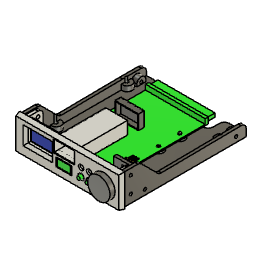
Gotek Case v24 (Autodesk Fusion 360 design; units mm, degrees)
Autodesk Fusion 360 part; units mm, degrees
(part 1 of 2)
sketch "Sketch1" plane through (0, 0, 0) normal (0, 0, 1) x (1, 0, 0)
  line L0 (-75, 0) -> (-75, 112)
  line L1 (-75, 112) -> (-134, 112)
  line L2 (-134, 112) -> (-134, 47.5)
  line L3 (-75, 0) -> (-114, 0)
  line L4 (-114, 0) -> (-114, 47.5)
  line L5 (-134, 47.5) -> (-114, 47.5)
  circle A0 centre (-79.5, 88.5) radius 1.5
  circle A1 centre (-129.5, 88.5) radius 1.5
  circle A2 centre (-79.5, 67.5) radius 1.5
  circle A3 centre (-129.5, 67.5) radius 1.5
  circle A4 centre (-79.5, 17.5) radius 1.5
  dimension "d1" = 112
  dimension "d2" = 59
  dimension "d3" = 64.5
  dimension "d4" = 39
  dimension "d11" = 3
  dimension "d12" = 3
  dimension "d13" = 3
  dimension "d14" = 3
  dimension "d15" = 3
  constraint vertical L0
  constraint perpendicular L0 L1
  constraint perpendicular L1 L2
  constraint perpendicular L0 L3
  constraint perpendicular L3 L4
  constraint perpendicular L4 L5
  measures "d1" distance of L0.start L0.end
  measures "d2" distance of L0.end L1.end
  measures "d3" distance of L1.end L2.end
  measures "d4" distance of L0.start L3.end
  measures "d11" diameter of A0
  measures "d12" diameter of A1
  measures "d13" diameter of A2
  measures "d14" diameter of A3
  measures "d15" diameter of A4
extrude "Extrude1" add sketch "Sketch1" along normal blind 1.1 makes body 1
box "BoxPrimitive1" add length 6 width 15 height 7 placed x (0, 1, 0) y (-1, 0, 0) z (0, 0, 1) at (-76, 2, 1.1) bodies 1
sketch "Sketch3" plane through (0, 2, 0) normal (0, -1, 0) x (1, 0, 0)
  line L0 (-91, 8.1) -> (-91, 1.1)
  line L1 (-91, 1.1) -> (-76, 1.1)
  line L2 (-76, 1.1) -> (-76, 8.1)
  line L3 (-76, 8.1) -> (-91, 8.1)
  circle A0 centre (-87.5, 5.1) radius 1.75
  circle A1 centre (-79.5, 5.1) radius 1.75
  dimension "d25" = 3.5
  dimension "d26" = 3.5
  measures "d25" diameter of A0
  measures "d26" diameter of A1
extrude "Extrude2" add sketch "Sketch3" along normal blind 5.5 contours A0 | A1 bodies 1
sketch "Sketch4" plane through (0, 0, 1.1) normal (0, 0, 1) x (-1, 0, 0)
  line L0 (76, -8) -> (76, -2)
  line L1 (76, -2) -> (91, -2)
  line L2 (91, -2) -> (91, -8)
  line L3 (91, -8) -> (76, -8)
  circle A0 centre (79.5, -88.5) radius 1.5
  circle A1 centre (129.5, -67.5) radius 1.5
  circle A2 centre (79.5, -67.5) radius 1.5
  circle A3 centre (129.5, -88.5) radius 1.5
  circle A4 centre (79.5, -17.5) radius 1.5
  line L4 (75, 0) -> (75, -112)
  line L5 (75, -112) -> (134, -112)
  line L6 (134, -112) -> (134, -47.5)
  line L7 (134, -47.5) -> (114, -47.5)
  line L8 (114, -47.5) -> (114, 0)
  line L9 (114, 0) -> (75, 0)
  line L10 (97.5, 1) -> (111.5, 1)
  line L11 (111.5, 1) -> (111.5, -13)
  line L12 (111.5, -13) -> (97.5, -13)
  line L13 (97.5, -13) -> (97.5, 1)
  dimension "d31" = 14
  dimension "d32" = 14
  constraint horizontal L10
  constraint vertical L11
  constraint horizontal L12
  constraint vertical L13
  measures "d31" distance of L10.start L10.end
  measures "d32" distance of L10.start L12.end
extrude "Extrude3" add sketch "Sketch4" along normal blind 8 contours L9 L10 L11 L13 | L9 L11 L12 L13 bodies 1
box "BoxPrimitive2" add length 3 width 59 height 5 placed x (0, -1, 0) y (1, 0, 0) z (0, 0, 1) at (-134, 112, 1.1) bodies 1
sketch "Sketch6" plane through (0, 112, 0) normal (0, 1, 0) x (-1, 0, 0)
  line L0 (75, 0) -> (134, 0)
  line L1 (134, 0) -> (134, 6.1)
  line L2 (134, 6.1) -> (75, 6.1)
  line L3 (75, 6.1) -> (75, 0)
  line L4 (76.25, 1.25) -> (132.75, 1.25)
  line L5 (132.75, 1.25) -> (132.75, 4.85)
  line L6 (132.75, 4.85) -> (76.25, 4.85)
  line L7 (76.25, 4.85) -> (76.25, 1.25)
  dimension "d40" = -1.25
extrude "Extrude4" add sketch "Sketch6" along normal blind 8 contours L4 L5 L6 L7 bodies 1
sketch "Sketch10" plane through (0, 0, 0) normal (0, 1, 0) x (1, 0, 0)
  line L0 (-200, -10) -> (-212, -10)
  line L1 (-212, -10) -> (-212, -24)
  line L2 (-212, -24) -> (-200, -24)
  line L3 (-200, -24) -> (-200, -10)
  dimension "d65" = 12
  dimension "d66" = 14
  constraint horizontal L0
  constraint vertical L1
  constraint horizontal L2
  constraint vertical L3
  measures "d65" distance of L0.start L0.end
  measures "d66" distance of L0.start L2.end
extrude "Extrude8" add sketch "Sketch10" along normal blind 6 separate body makes body 2
cylinder "CylinderPrimitive1" add diameter 7 height 7.5 placed x (1, 0, 0) y (0, 0, 1) z (0, -1, 0) at (-206, 0, 17) bodies 2
cylinder "CylinderPrimitive2" add diameter 4 height 1 placed x (1, 0, 0) y (0, 0, 1) z (0, -1, 0) at (-206, -7.5, 17) bodies 2
cylinder "CylinderPrimitive3" add diameter 6 height 12.5 placed x (1, 0, 0) y (0, 0, 1) z (0, -1, 0) at (-206, -8.5, 17) bodies 2
sketch "Sketch14" plane through (0, -21, 0) normal (0, -1, 0) x (1, 0, 0)
  circle A0 centre (-206, 17) radius 3
  line L0 (-209.5054, 18.5) -> (-202.5, 18.5)
  line L1 (-202.5, 18.5) -> (-202.5, 20.3)
  line L2 (-202.5, 20.3) -> (-209.5054, 20.3)
  line L3 (-209.5054, 20.3) -> (-209.5054, 18.5)
  constraint horizontal L0
  constraint vertical L1
  constraint horizontal L2
  constraint vertical L3
extrude "Extrude9" cut sketch "Sketch14" against normal blind 12 contours A0 L0 | A0 L0 L1 L2 L3 picked at (-205.8141, 19.2331) bodies 2
sketch "Sketch15" plane through (0, 0, 24) normal (0, 0, 1) x (-1, 0, 0)
  line L0 (212, 0) -> (200, 0)
  line L1 (200, 0) -> (200, -6)
  line L2 (200, -6) -> (212, -6)
  line L3 (212, -6) -> (212, 0)
  line L4 (209.29, -6) -> (207.79, -6)
  line L5 (207.79, -6) -> (207.79, -3)
  line L6 (207.79, -3) -> (209.29, -3)
  line L7 (209.29, -3) -> (209.29, -6)
  line L8 (209.29, -6) -> (207.79, -3) construction
  line L9 (207.79, -6) -> (209.29, -3) construction
  line L10 (202.71, -6) -> (204.21, -6)
  line L11 (204.21, -6) -> (204.21, -3)
  line L12 (204.21, -3) -> (202.71, -3)
  line L13 (202.71, -3) -> (202.71, -6)
  line L14 (202.71, -6) -> (204.21, -3) construction
  line L15 (204.21, -6) -> (202.71, -3) construction
  line L16 (206.75, -6) -> (205.25, -6)
  line L17 (205.25, -6) -> (205.25, -3)
  line L18 (205.25, -3) -> (206.75, -3)
  line L19 (206.75, -3) -> (206.75, -6)
  line L20 (206.75, -6) -> (205.25, -3) construction
  line L21 (205.25, -6) -> (206.75, -3) construction
  point P0 (208.54, -4.5)
  point P1 (203.46, -4.5)
  point P2 (206, -4.5)
  dimension "d82" = 1.5
  dimension "d83" = 1.5
  dimension "d84" = 1.5
  constraint horizontal L4
  constraint perpendicular L4 L5
  constraint parallel L4 L6
  constraint parallel L5 L7
  constraint coincident L8 P0
  constraint coincident L9 P0
  constraint horizontal L10
  constraint perpendicular L10 L11
  constraint parallel L10 L12
  constraint parallel L11 L13
  constraint coincident L14 P1
  constraint coincident L15 P1
  constraint horizontal L16
  constraint perpendicular L16 L17
  constraint parallel L16 L18
  constraint parallel L17 L19
  constraint coincident L20 P2
  constraint coincident L21 P2
  measures "d82" distance of L5.end L6.end
  measures "d83" distance of L11.end L12.end
  measures "d84" distance of L17.end L18.end
extrude "Extrude10" add sketch "Sketch15" along normal blind 1.5 contours L2 L4 L5 L6 L7 | L2 L10 L11 L12 L13 | L2 L16 L17 L18 L19 bodies 2
sketch "Sketch16" plane through (0, 6, 0) normal (0, 1, 0) x (-1, 0, 0)
  line L0 (200, 24) -> (200, 10)
  line L1 (200, 10) -> (212, 10)
  line L2 (212, 10) -> (212, 24)
  line L3 (212, 24) -> (209.29, 24)
  line L4 (209.29, 24) -> (209.29, 25.5)
  line L5 (209.29, 25.5) -> (207.79, 25.5)
  line L6 (207.79, 25.5) -> (207.79, 24)
  line L7 (207.79, 24) -> (206.75, 24)
  line L8 (206.75, 24) -> (206.75, 25.5)
  line L9 (206.75, 25.5) -> (205.25, 25.5)
  line L10 (205.25, 25.5) -> (205.25, 24)
  line L11 (205.25, 24) -> (204.21, 24)
  line L12 (204.21, 24) -> (204.21, 25.5)
  line L13 (204.21, 25.5) -> (202.71, 25.5)
  line L14 (202.71, 25.5) -> (202.71, 24)
  line L15 (202.71, 24) -> (200, 24)
  line L16 (203.96, 25.5) -> (202.96, 25.5)
  line L17 (202.96, 25.5) -> (202.96, 25.2)
  line L18 (202.96, 25.2) -> (203.96, 25.2)
  line L19 (203.96, 25.2) -> (203.96, 25.5)
  line L20 (203.96, 25.5) -> (202.96, 25.2) construction
  line L21 (202.96, 25.5) -> (203.96, 25.2) construction
  line L22 (205.5, 25.5) -> (206.5, 25.5)
  line L23 (206.5, 25.5) -> (206.5, 25.2)
  line L24 (206.5, 25.2) -> (205.5, 25.2)
  line L25 (205.5, 25.2) -> (205.5, 25.5)
  line L26 (205.5, 25.5) -> (206.5, 25.2) construction
  line L27 (206.5, 25.5) -> (205.5, 25.2) construction
  line L28 (208.04, 25.5) -> (209.04, 25.5)
  line L29 (209.04, 25.5) -> (209.04, 25.2)
  line L30 (209.04, 25.2) -> (208.04, 25.2)
  line L31 (208.04, 25.2) -> (208.04, 25.5)
  line L32 (208.04, 25.5) -> (209.04, 25.2) construction
  line L33 (209.04, 25.5) -> (208.04, 25.2) construction
  point P0 (203.46, 25.35)
  point P1 (206, 25.35)
  point P2 (208.54, 25.35)
  dimension "d90" = 1
  dimension "d91" = 1
  dimension "d92" = 1
  constraint horizontal L16
  constraint perpendicular L16 L17
  constraint parallel L16 L18
  constraint parallel L17 L19
  constraint coincident L20 P0
  constraint coincident L21 P0
  constraint horizontal L22
  constraint perpendicular L22 L23
  constraint parallel L22 L24
  constraint parallel L23 L25
  constraint coincident L26 P1
  constraint coincident L27 P1
  constraint horizontal L28
  constraint perpendicular L28 L29
  constraint parallel L28 L30
  constraint parallel L29 L31
  constraint coincident L32 P2
  constraint coincident L33 P2
  measures "d90" distance of L17.end L18.end
  measures "d91" distance of L23.end L24.end
  measures "d92" distance of L29.end L30.end
extrude "Extrude11" add sketch "Sketch16" along normal blind 4 contours L13 L16 L17 L18 L19 | L5 L28 L29 L30 L31 | L9 L22 L23 L24 L25 bodies 2
box "BoxPrimitive3" add length 1 width 1 height 1 placed x (0, 0, -1) y (1, 0, 0) z (0, -1, 0) at (-206, 0, 24) bodies 2
box "BoxPrimitive4" add length 1 width 1 height 1 placed x (0, 0, -1) y (1, 0, 0) z (0, -1, 0) at (-207, 0, 24) bodies 2
sketch "Sketch19" plane through (0, 6, 0) normal (0, 1, 0) x (-1, 0, 0)
  line L0 (209.04, 25.5) -> (209.04, 25.2)
  line L1 (209.04, 25.2) -> (208.04, 25.2)
  line L2 (208.04, 25.2) -> (208.04, 25.5)
  line L3 (208.04, 25.5) -> (207.79, 25.5)
  line L4 (207.79, 25.5) -> (207.79, 24)
  line L5 (207.79, 24) -> (206.75, 24)
  line L6 (206.75, 24) -> (206.75, 25.5)
  line L7 (206.75, 25.5) -> (206.5, 25.5)
  line L8 (206.5, 25.5) -> (206.5, 25.2)
  line L9 (206.5, 25.2) -> (205.5, 25.2)
  line L10 (205.5, 25.2) -> (205.5, 25.5)
  line L11 (205.5, 25.5) -> (205.25, 25.5)
  line L12 (205.25, 25.5) -> (205.25, 24)
  line L13 (205.25, 24) -> (204.21, 24)
  line L14 (204.21, 24) -> (204.21, 25.5)
  line L15 (204.21, 25.5) -> (203.96, 25.5)
  line L16 (203.96, 25.5) -> (203.96, 25.2)
  line L17 (203.96, 25.2) -> (202.96, 25.2)
  line L18 (202.96, 25.2) -> (202.96, 25.5)
  line L19 (202.96, 25.5) -> (202.71, 25.5)
  line L20 (202.71, 25.5) -> (202.71, 24)
  line L21 (202.71, 24) -> (200, 24)
  line L22 (200, 24) -> (200, 10)
  line L23 (200, 10) -> (212, 10)
  line L24 (212, 10) -> (212, 24)
  line L25 (212, 24) -> (209.29, 24)
  line L26 (209.29, 24) -> (209.29, 25.5)
  line L27 (209.29, 25.5) -> (209.04, 25.5)
  line L28 (208.04, 10) -> (209.04, 10)
  line L29 (209.04, 10) -> (209.04, 10.3)
  line L30 (209.04, 10.3) -> (208.04, 10.3)
  line L31 (208.04, 10.3) -> (208.04, 10)
  line L32 (208.04, 10) -> (209.04, 10.3) construction
  line L33 (209.04, 10) -> (208.04, 10.3) construction
  line L34 (203.96, 10) -> (202.96, 10)
  line L35 (202.96, 10) -> (202.96, 10.3)
  line L36 (202.96, 10.3) -> (203.96, 10.3)
  line L37 (203.96, 10.3) -> (203.96, 10)
  line L38 (203.96, 10) -> (202.96, 10.3) construction
  line L39 (202.96, 10) -> (203.96, 10.3) construction
  point P0 (208.54, 10.15)
  point P1 (203.46, 10.15)
  dimension "d106" = 1
  dimension "d107" = 1
  constraint horizontal L28
  constraint perpendicular L28 L29
  constraint parallel L28 L30
  constraint parallel L29 L31
  constraint coincident L32 P0
  constraint coincident L33 P0
  constraint horizontal L34
  constraint perpendicular L34 L35
  constraint parallel L34 L36
  constraint parallel L35 L37
  constraint coincident L38 P1
  constraint coincident L39 P1
  measures "d106" distance of L29.end L30.end
  measures "d107" distance of L35.end L36.end
extrude "Extrude12" add sketch "Sketch19" along normal blind 4 contours L23 L28 L29 L30 L31 | L23 L34 L35 L36 L37 bodies 2
sketch "Sketch20" plane through (0, 6, 0) normal (0, 1, 0) x (-1, 0, 0)
  line L0 (202.96, 10) -> (202.96, 10.3)
  line L1 (202.96, 10.3) -> (203.96, 10.3)
  line L2 (203.96, 10.3) -> (203.96, 10)
  line L3 (203.96, 10) -> (208.04, 10)
  line L4 (208.04, 10) -> (208.04, 10.3)
  line L5 (208.04, 10.3) -> (209.04, 10.3)
  line L6 (209.04, 10.3) -> (209.04, 10)
  line L7 (209.04, 10) -> (212, 10)
  line L8 (212, 10) -> (212, 24)
  line L9 (212, 24) -> (209.29, 24)
  line L10 (209.29, 24) -> (209.29, 25.5)
  line L11 (209.29, 25.5) -> (209.04, 25.5)
  line L12 (209.04, 25.5) -> (209.04, 25.2)
  line L13 (209.04, 25.2) -> (208.04, 25.2)
  line L14 (208.04, 25.2) -> (208.04, 25.5)
  line L15 (208.04, 25.5) -> (207.79, 25.5)
  line L16 (207.79, 25.5) -> (207.79, 24)
  line L17 (207.79, 24) -> (206.75, 24)
  line L18 (206.75, 24) -> (206.75, 25.5)
  line L19 (206.75, 25.5) -> (206.5, 25.5)
  line L20 (206.5, 25.5) -> (206.5, 25.2)
  line L21 (206.5, 25.2) -> (205.5, 25.2)
  line L22 (205.5, 25.2) -> (205.5, 25.5)
  line L23 (205.5, 25.5) -> (205.25, 25.5)
  line L24 (205.25, 25.5) -> (205.25, 24)
  line L25 (205.25, 24) -> (204.21, 24)
  line L26 (204.21, 24) -> (204.21, 25.5)
  line L27 (204.21, 25.5) -> (203.96, 25.5)
  line L28 (203.96, 25.5) -> (203.96, 25.2)
  line L29 (203.96, 25.2) -> (202.96, 25.2)
  line L30 (202.96, 25.2) -> (202.96, 25.5)
  line L31 (202.96, 25.5) -> (202.71, 25.5)
  line L32 (202.71, 25.5) -> (202.71, 24)
  line L33 (202.71, 24) -> (200, 24)
  line L34 (200, 24) -> (200, 10)
  line L35 (200, 10) -> (202.96, 10)
  line L36 (200, 17) -> (200, 17)
  line L37 (200, 18) -> (202, 18)
  line L38 (202, 18) -> (202, 16)
  line L39 (202, 16) -> (200, 16)
  line L40 (200, 16) -> (200, 18)
  line L41 (200, 18) -> (202, 16) construction
  line L42 (202, 18) -> (200, 16) construction
  line L43 (212, 18) -> (210, 18)
  line L44 (210, 18) -> (210, 16)
  line L45 (210, 16) -> (212, 16)
  line L46 (212, 16) -> (212, 18)
  line L47 (212, 18) -> (210, 16) construction
  line L48 (210, 18) -> (212, 16) construction
  point P0 (201, 17)
  point P1 (211, 17)
  constraint midpoint L34 L36.start
  constraint perpendicular L34 L36
  constraint horizontal L37
  constraint perpendicular L37 L38
  constraint parallel L37 L39
  constraint parallel L38 L40
  constraint coincident L34 L37.start
  constraint coincident L41 P0
  constraint coincident L42 P0
  constraint horizontal L43
  constraint perpendicular L43 L44
  constraint parallel L43 L45
  constraint parallel L44 L46
  constraint coincident L8 L43.start
  constraint coincident L47 P1
  constraint coincident L48 P1
extrude "Extrude13" add sketch "Sketch20" along normal blind 4 contours L34 L37 L38 L39 L40 | L8 L43 L44 L45 L46 bodies 2
thread "Thread1" "ISO Metric profile 7.0 M7x1 6g" major diameter 6.884 minor diameter 5.744 pitch 1 angle 60 modelled right hand crest width 0.1446 on face at (-203.5562, -5, 19.5055) crest through (-202.558, 0.25, 17) on bodies 2
sketch "Sketch61" plane through (0, -1, 0) normal (0, -1, 0) x (1, 0, 0)
  line L0 (-111.5, 1.1) -> (-97.5, 1.1)
  line L1 (-97.5, 1.1) -> (-97.5, 9.1)
  line L2 (-97.5, 9.1) -> (-111.5, 9.1)
  line L3 (-111.5, 9.1) -> (-111.5, 1.1)
  line L4 (-111, 2.1) -> (-98, 2.1)
  line L5 (-98, 2.1) -> (-98, 9.1)
  line L6 (-98, 9.1) -> (-111, 9.1)
  line L7 (-111, 9.1) -> (-111, 2.1)
  dimension "d304" = 13
  dimension "d305" = 7
  constraint horizontal L4
  constraint vertical L5
  constraint horizontal L6
  constraint vertical L7
  measures "d304" distance of L4.start L4.end
  measures "d305" distance of L4.start L6.end
extrude "Extrude40" cut sketch "Sketch61" against normal blind 10 contours L0 L1 L2 L3 L4 L5 L7 bodies 1
sketch "Sketch62" plane through (0, 0, 0) normal (0, 1, 0) x (1, 0, 0)
  line L0 (-142.5, -5) -> (-142.5, -32.8)
  line L1 (-142.5, -32.8) -> (-170, -32.8)
  line L2 (-170, -32.8) -> (-170, -5)
  line L3 (-149.5, -5) -> (-149.5, -7) construction
  line L4 (-149.5, -7) -> (-163, -7) construction
  line L5 (-163, -7) -> (-163, -5) construction
  line L6 (-163, -5) -> (-163, -7)
  line L7 (-149.5, -5) -> (-149.5, -7)
  line L8 (-163, -7) -> (-149.5, -7)
  line L9 (-170, -5) -> (-163, -5)
  line L10 (-149.5, -5) -> (-142.5, -5)
  circle A0 centre (-168, -30.8) radius 1
  circle A1 centre (-144.5, -30.8) radius 1
  circle A2 centre (-168, -7) radius 1
  circle A3 centre (-144.5, -7) radius 1
  dimension "d308" = 27.5
  dimension "d309" = 27.8
  dimension "d312" = 2
  dimension "d314" = 2
  dimension "d315" = 2
  dimension "d316" = 2
  dimension "d317" = 2
  constraint horizontal L9
  constraint vertical L0
  constraint horizontal L1
  constraint vertical L2
  constraint vertical L3
  constraint horizontal L4
  constraint vertical L5
  constraint collinear L9 L10
  measures "d308" distance of L2.end L0.start
  measures "d309" distance of L2.end L1.end
  measures "d312" distance of L5.end L4.end
  measures "d314" diameter of A0
  measures "d315" diameter of A1
  measures "d316" diameter of A2
  measures "d317" diameter of A3
extrude "Extrude41" add sketch "Sketch62" along normal blind 1 separate body makes body 3
sketch "Sketch63" plane through (0, 0, 0) normal (0, -1, 0) x (1, 0, 0)
  circle A0 centre (-168, 30.8) radius 1
  circle A1 centre (-144.5, 7) radius 1
  circle A2 centre (-168, 7) radius 1
  circle A3 centre (-144.5, 30.8) radius 1
  line L0 (-149.5, 7) -> (-149.5, 5)
  line L1 (-149.5, 5) -> (-142.5, 5)
  line L2 (-142.5, 5) -> (-142.5, 32.8)
  line L3 (-142.5, 32.8) -> (-170, 32.8)
  line L4 (-170, 32.8) -> (-170, 5)
  line L5 (-170, 5) -> (-163, 5)
  line L6 (-163, 5) -> (-163, 7)
  line L7 (-163, 7) -> (-149.5, 7)
  line L8 (-170, 32.8) -> (-170, 28.53) construction
  line L9 (-170, 28.53) -> (-142.5, 28.53)
  line L10 (-142.5, 28.53) -> (-142.5, 9.27)
  line L11 (-142.5, 9.27) -> (-170, 9.27)
  line L12 (-170, 9.27) -> (-170, 28.53)
  dimension "d320" = 4.27
  dimension "d321" = 27.5
  dimension "d322" = 19.26
  constraint coincident L3.end L4.start
  constraint perpendicular L3 L8
  constraint horizontal L9
  constraint vertical L10
  constraint horizontal L11
  constraint vertical L12
  measures "d320" distance of L3.end L8.end
  measures "d321" distance of L8.end L9.end
  measures "d322" distance of L8.end L11.end
extrude "Extrude42" add sketch "Sketch63" along normal blind 1.7 contours L2 L4 L9 L10 L11 L12 bodies 3
sketch "Sketch64" plane through (0, -1.7, 0) normal (0, -1, 0) x (1, 0, 0)
  line L0 (-170, 9.27) -> (-142.5, 9.27)
  line L1 (-142.5, 9.27) -> (-142.5, 28.53)
  line L2 (-142.5, 28.53) -> (-170, 28.53)
  line L3 (-170, 28.53) -> (-170, 9.27)
  line L4 (-170, 28.53) -> (-142.5, 28.53) construction
  line L5 (-142.5, 28.53) -> (-142.5, 32.8) construction
  line L6 (-142.5, 32.8) -> (-170, 32.8) construction
  line L7 (-170, 32.8) -> (-170, 28.53) construction
  circle A0 centre (-168, 30.8) radius 1 construction
  circle A1 centre (-144.5, 30.8) radius 1 construction
  line L8 (-156.25, 32.8) -> (-156.25, 27.43) construction
  line L9 (-156.25, 27.43) -> (-156.25, 20.998) construction
  line L10 (-168.25, 27.498) -> (-144.25, 27.498)
  line L11 (-144.25, 27.498) -> (-144.25, 14.498)
  line L12 (-144.25, 14.498) -> (-168.25, 14.498)
  line L13 (-168.25, 14.498) -> (-168.25, 27.498)
  line L14 (-168.25, 27.498) -> (-144.25, 14.498) construction
  line L15 (-144.25, 27.498) -> (-168.25, 14.498) construction
  point P0 (-156.25, 20.998)
  dimension "d325" = 5.37
  dimension "d326" = 6.432
  dimension "d327" = 24
  dimension "d328" = 13
  constraint midpoint L6 L8.start
  constraint perpendicular L6 L8
  constraint perpendicular L2 L9
  constraint horizontal L10
  constraint perpendicular L10 L11
  constraint parallel L10 L12
  constraint parallel L11 L13
  constraint coincident L14 P0
  constraint coincident L15 P0
  constraint coincident P0 L9.end
  measures "d325" distance of L8.start L8.end
  measures "d326" distance of L8.end P0
  measures "d327" distance of L11.end L12.end
  measures "d328" distance of L10.end L11.end
extrude "Extrude43" cut sketch "Sketch64" against normal blind 0.25 contours L10 L11 L12 L13 bodies 3
sketch "Front Panel 1" plane through (0, 0, 0) normal (0, 1, 0) x (1, 0, 0)
  line L0 (-1, 1) -> (102.6, 1)
  line L1 (102.6, 1) -> (102.6, -31)
  line L2 (102.6, -31) -> (-1, -31)
  line L3 (-1, -31) -> (-1, 1)
extrude "Extrude44" add sketch "Front Panel 1" against normal blind 5 separate body makes body 4
chamfer "Chamfer9" distance 1 distance2 5 4 edges at (50.8, -5, 31) (102.6, -5, 15) (50.8, -5, -1) (-1, -5, 15) measured on face at (33.5333, -5, 20.3333) measured on face at (33.5333, -5, 20.3333) measured on face at (33.5333, -5, 20.3333) measured on face at (33.5333, -5, 20.3333) on bodies 4
sketch "FP Lugs" plane through (0, 0, 0) normal (0, 1, 0) x (-1, 0, 0)
  line L0 (1, 31) -> (-102.6, 31)
  line L1 (-102.6, 31) -> (-102.6, -1)
  line L2 (-102.6, -1) -> (1, -1)
  line L3 (1, -1) -> (1, 31)
  line L4 (-99.6, 20) -> (-94.6, 20)
  line L5 (-94.6, 20) -> (-94.6, 10)
  line L6 (-94.6, 10) -> (-99.6, 10)
  line L7 (-99.6, 10) -> (-99.6, 20)
  line L8 (-99.6, 20) -> (-94.6, 10) construction
  line L9 (-94.6, 20) -> (-99.6, 10) construction
  line L10 (-2, 10) -> (-7, 10)
  line L11 (-7, 10) -> (-7, 20)
  line L12 (-7, 20) -> (-2, 20)
  line L13 (-2, 20) -> (-2, 10)
  line L14 (-2, 10) -> (-7, 20) construction
  line L15 (-7, 10) -> (-2, 20) construction
  point P0 (-97.1, 15)
  point P1 (-4.5, 15)
  dimension "d342" = 5
  dimension "d343" = 10
  dimension "d344" = 5
  dimension "d345" = 10
  constraint horizontal L4
  constraint perpendicular L4 L5
  constraint parallel L4 L6
  constraint parallel L5 L7
  constraint coincident L8 P0
  constraint coincident L9 P0
  constraint horizontal L10
  constraint perpendicular L10 L11
  constraint parallel L10 L12
  constraint parallel L11 L13
  constraint coincident L14 P1
  constraint coincident L15 P1
  measures "d342" distance of L5.end L6.end
  measures "d343" distance of L4.end L5.end
  measures "d344" distance of L11.end L12.end
  measures "d345" distance of L10.end L11.end
extrude "Extrude45" add sketch "FP Lugs" along normal blind 10 contours L4 L5 L6 L7 | L10 L11 L12 L13 bodies 4
sketch "OLED Supp" plane through (99.6, 0, 0) normal (1, 0, 0) x (0, 1, 0)
  line L0 (0, 20) -> (0, 10)
  line L1 (0, 10) -> (10, 10)
  line L2 (10, 10) -> (10, 20)
  line L3 (10, 20) -> (0, 20)
  circle A0 centre (5, 15) radius 1.75
  dimension "d348" = 3.5
  measures "d348" diameter of A0
extrude "Extrude46" cut sketch "OLED Supp" against normal blind 110 contours A0 bodies 4
hole "Hole7" at (7, 5, 15) direction (-1, 0, 0) diameter 6 depth 3 tip angle 180 bodies 4
hole "Hole8" at (94.6, 5, 15) direction (1, 0, 0) diameter 6 depth 3 tip angle 180 bodies 4
fillet "Fillet2" radius 5 4 edges at (4.5, 10, 10) (97.1, 10, 10) (97.1, 10, 20) (4.5, 10, 20) on bodies 4
move_body "Move13" bodies 3 to x (1, 0, 0) y (0, 1, 0) z (0, 0, 1) at (178, 2, -4)
move_body "Move14" bodies 3 to x (1, 0, 0) y (0, 1, 0) z (0, 0, 1) at (0, 0, 0.06)
sketch "OLED Fix" plane through (0, 0, 0) normal (0, 1, 0) x (-1, 0, 0)
  line L0 (-2, 20) -> (-2, 10)
  line L1 (-2, 10) -> (-7, 10)
  line L2 (-7, 10) -> (-7, 20)
  line L3 (-7, 20) -> (-2, 20)
  line L4 (-99.6, 10) -> (-99.6, 20)
  line L5 (-99.6, 20) -> (-94.6, 20)
  line L6 (-94.6, 20) -> (-94.6, 10)
  line L7 (-94.6, 10) -> (-99.6, 10)
  line L8 (1, 31) -> (-102.6, 31)
  line L9 (-102.6, 31) -> (-102.6, -1)
  line L10 (-102.6, -1) -> (1, -1)
  line L11 (1, -1) -> (1, 31)
  circle A0 centre (-33.5, 26.86) radius 1.5
  circle A1 centre (-33.5, 3.06) radius 1.5
  circle A2 centre (-10, 26.86) radius 1.5
  circle A3 centre (-10, 3.06) radius 1.5
  dimension "d359" = 3
  dimension "d360" = 3
  dimension "d361" = 3
  dimension "d362" = 3
  measures "d359" diameter of A0
  measures "d360" diameter of A1
  measures "d361" diameter of A2
  measures "d362" diameter of A3
extrude "Extrude47" add sketch "OLED Fix" along normal blind 2 contours A0 | A1 | A2 | A3 bodies 4
cylinder "CylinderPrimitive11" add diameter 1.9 height 3 placed x (1, 0, 0) y (0, 0, -1) z (0, 1, 0) at (33.5, 2, 26.86) bodies 4
cylinder "CylinderPrimitive12" add diameter 1.9 height 3 placed x (1, 0, 0) y (0, 0, -1) z (0, 1, 0) at (10, 2, 26.86) bodies 4
cylinder "CylinderPrimitive13" add diameter 1.9 height 3 placed x (1, 0, 0) y (0, 0, -1) z (0, 1, 0) at (10, 2, 3.06) bodies 4
cylinder "CylinderPrimitive14" add diameter 1.9 height 3 placed x (1, 0, 0) y (0, 0, -1) z (0, 1, 0) at (33.5, 2, 3.06) bodies 4
sketch "OLED Window" plane through (0, 0, 0) normal (0, 1, 0) x (-1, 0, 0)
  line L0 (0, 0) -> (-101.6, 0)
  line L1 (-101.6, 0) -> (-101.6, 30)
  line L2 (-101.6, 30) -> (0, 30)
  line L3 (0, 30) -> (0, 0)
  line L4 (-33.75, 23.558) -> (-33.75, 10.558)
  line L5 (-33.75, 10.558) -> (-9.75, 10.558)
  line L6 (-9.75, 10.558) -> (-9.75, 23.558)
  line L7 (-9.75, 23.558) -> (-33.75, 23.558)
  line L8 (-9.75, 23.558) -> (-33.75, 23.558)
  line L9 (-33.75, 23.558) -> (-33.75, 10.558)
  line L10 (-33.75, 10.558) -> (-9.75, 10.558)
  line L11 (-9.75, 10.558) -> (-9.75, 23.558)
  line L12 (-33.75, 10.558) -> (-9.75, 10.558)
  line L13 (-9.75, 10.558) -> (-9.75, 23.558)
  line L14 (-9.75, 23.558) -> (-33.75, 23.558)
  line L15 (-33.75, 23.558) -> (-33.75, 10.558)
  constraint horizontal L8
  constraint vertical L9
  constraint horizontal L10
  constraint vertical L11
  constraint coincident L4.end L5.start
  constraint coincident L6.end L7.start
  constraint horizontal L12
  constraint vertical L13
  constraint horizontal L14
  constraint vertical L15
extrude "Extrude48" cut sketch "OLED Window" against normal blind 5 contours L4 L5 L6 L7 L8 L9 L10 L11 L12 L13 L14 L15 bodies 4
chamfer "Chamfer10" distance 2.5 angle 45 4 edges at (21.75, -5, 10.558) (9.75, -5, 17.058) (21.75, -5, 23.558) (33.75, -5, 17.058) on bodies 4
move_body "Move15" bodies 1 to x (1, 0, 0) y (0, 1, 0) z (0, 0, 1) at (150, -4, 5)
move_body "Move16" bodies 1 to x (1, 0, 0) y (0, 1, 0) z (0, 0, 1) at (2, 0, 0)
move_body "Move17" bodies 2 to x (1, 0, 0) y (0, 1, 0) z (0, 0, 1) at (292, 0, 0)
move_body "Move18" bodies 2 to x (1, 0, 0) y (0, 1, 0) z (0, 0, 1) at (2, 0, -2)
move_body "Move19" bodies 2 to x (1, 0, 0) y (0, 1, 0) z (0, 0, 1) at (0, 16, 0)
sketch "PCB Cutout" plane through (0, 0, 0) normal (0, 1, 0) x (-1, 0, 0)
  line L0 (-9.75, 10.558) -> (-33.75, 10.558)
  line L1 (-33.75, 10.558) -> (-33.75, 23.558)
  line L2 (-33.75, 23.558) -> (-9.75, 23.558)
  line L3 (-9.75, 23.558) -> (-9.75, 10.558)
  circle A0 centre (-33.5, 3.06) radius 1.5
  circle A1 centre (-33.5, 26.86) radius 1.5
  circle A2 centre (-10, 3.06) radius 1.5
  circle A3 centre (-10, 26.86) radius 1.5
  line L4 (-2, 20) -> (-2, 10)
  line L5 (-2, 10) -> (-7, 10)
  line L6 (-7, 10) -> (-7, 20)
  line L7 (-7, 20) -> (-2, 20)
  line L8 (-99.6, 10) -> (-99.6, 20)
  line L9 (-99.6, 20) -> (-94.6, 20)
  line L10 (-94.6, 20) -> (-94.6, 10)
  line L11 (-94.6, 10) -> (-99.6, 10)
  line L12 (1, 31) -> (-102.6, 31)
  line L13 (-102.6, 31) -> (-102.6, -1)
  line L14 (-102.6, -1) -> (1, -1)
  line L15 (1, -1) -> (1, 31)
  line L16 (-37, 3) -> (-81, 3)
  line L17 (-81, 3) -> (-81, 16)
  line L18 (-81, 16) -> (-37, 16)
  line L19 (-37, 16) -> (-37, 3)
  constraint horizontal L16
  constraint vertical L17
  constraint horizontal L18
  constraint vertical L19
extrude "Extrude49" cut sketch "PCB Cutout" against normal blind 4 contours L16 L17 L18 L19 bodies 4
sketch "Gotek Holes" plane through (0, -5, 0) normal (0, -1, 0) x (1, 0, 0)
  line L0 (0, 0) -> (101.6, 0)
  line L1 (101.6, 0) -> (101.6, 30)
  line L2 (101.6, 30) -> (0, 30)
  line L3 (0, 30) -> (0, 0)
  line L4 (36.25, 8.058) -> (7.25, 8.058)
  line L5 (7.25, 8.058) -> (7.25, 26.058)
  line L6 (7.25, 26.058) -> (36.25, 26.058)
  line L7 (36.25, 26.058) -> (36.25, 8.058)
  line L8 (54.75, 14.35) -> (40.25, 14.35)
  line L9 (40.25, 14.35) -> (40.25, 6.85)
  line L10 (40.25, 6.85) -> (54.75, 6.85)
  line L11 (54.75, 6.85) -> (54.75, 14.35)
  circle A0 centre (64.5, 10.1) radius 2
  circle A1 centre (72.5, 10.1) radius 2
  circle A2 centre (72.5, 18.1) radius 1.625
  dimension "d381" = 8
  dimension "d382" = 3.25
  measures "d381" distance of A1.centre A2.centre
  measures "d382" diameter of A2
extrude "Extrude50" cut sketch "Gotek Holes" against normal blind 5 contours L8 L9 L10 L11 | A0 | A1 | A2 bodies 4
chamfer "Chamfer11" distance 1 angle 45 3 edges at (62.6353, -5, 10.8232) (70.6353, -5, 10.8232) (70.985, -5, 18.6876) on bodies 4
sketch "Encoder hole" plane through (0, -5, 0) normal (0, -1, 0) x (1, 0, 0)
  circle A0 centre (72.5, 10.1) radius 3
  line L0 (36.25, 8.058) -> (7.25, 8.058)
  line L1 (7.25, 8.058) -> (7.25, 26.058)
  line L2 (7.25, 26.058) -> (36.25, 26.058)
  line L3 (36.25, 26.058) -> (36.25, 8.058)
  line L4 (0, 0) -> (101.6, 0)
  line L5 (101.6, 0) -> (101.6, 30)
  line L6 (101.6, 30) -> (0, 30)
  line L7 (0, 30) -> (0, 0)
  line L8 (40.25, 14.35) -> (54.75, 14.35)
  line L9 (54.75, 14.35) -> (54.75, 6.85)
  line L10 (54.75, 6.85) -> (40.25, 6.85)
  line L11 (40.25, 6.85) -> (40.25, 14.35)
  circle A1 centre (64.5, 10.1) radius 3
  circle A2 centre (72.5, 18.1) radius 2.625
  circle A3 centre (88, 15) radius 7
  dimension "d386" = 14
  measures "d386" diameter of A3
extrude "Extrude51" cut sketch "Encoder hole" against normal blind 5 contours A3 bodies 4
sketch "USB Hole" plane through (0, -5, 0) normal (0, -1, 0) x (1, 0, 0)
  circle A0 centre (88, 15) radius 7
  circle A1 centre (72.5, 10.1) radius 3
  line L0 (36.25, 8.058) -> (7.25, 8.058)
  line L1 (7.25, 8.058) -> (7.25, 26.058)
  line L2 (7.25, 26.058) -> (36.25, 26.058)
  line L3 (36.25, 26.058) -> (36.25, 8.058)
  line L4 (0, 0) -> (101.6, 0)
  line L5 (101.6, 0) -> (101.6, 30)
  line L6 (101.6, 30) -> (0, 30)
  line L7 (0, 30) -> (0, 0)
  line L8 (40.25, 14.35) -> (54.75, 14.35)
  line L9 (54.75, 14.35) -> (54.75, 6.85)
  line L10 (54.75, 6.85) -> (40.25, 6.85)
  line L11 (40.25, 6.85) -> (40.25, 14.35)
  circle A2 centre (64.5, 10.1) radius 3
  circle A3 centre (72.5, 18.1) radius 2.625
  line L12 (47.5, 14.35) -> (47.5, 16)
  line L13 (58, 17) -> (37, 29) construction
  line L14 (37, 17) -> (58, 29) construction
  line L15 (57.5, 17.5) -> (37.5, 17.5)
  line L16 (37.5, 17.5) -> (37.5, 28.5)
  line L17 (37.5, 28.5) -> (57.5, 28.5)
  line L18 (57.5, 28.5) -> (57.5, 17.5)
  line L19 (57.5, 17.5) -> (37.5, 28.5) construction
  line L20 (37.5, 17.5) -> (57.5, 28.5) construction
  point P0 (47.5, 23)
  point P1 (47.5, 23)
  dimension "d389" = 7
  dimension "d390" = 20
  dimension "d391" = 11
  constraint midpoint L8 L12.start
  constraint perpendicular L8 L12
  constraint coincident L13 P1
  constraint coincident L14 P1
  constraint horizontal L15
  constraint perpendicular L15 L16
  constraint parallel L15 L17
  constraint parallel L16 L18
  constraint coincident L19 P1
  constraint coincident L20 P1
  constraint coincident P1 P0
  measures "d389" distance of L12.end P1
  measures "d390" distance of L16.end L17.end
  measures "d391" distance of L15.end L16.end
extrude "Extrude52" cut sketch "USB Hole" against normal blind 5 contours L15 L16 L17 L18 bodies 4
sketch "USB Holder" plane through (0, 0, 0) normal (0, 1, 0) x (-1, 0, 0)
  line L0 (-37.5, 28.5) -> (-37.5, 17.5)
  line L1 (-37.5, 17.5) -> (-57.5, 17.5)
  line L2 (-57.5, 17.5) -> (-57.5, 28.5)
  line L3 (-57.5, 28.5) -> (-37.5, 28.5)
  arc A0 (-94.6, 12.6676) -> (-81, 15) centre (-88, 15) ccw
  line L4 (-94.6, 12.6676) -> (-94.6, 10)
  line L5 (-94.6, 10) -> (-99.6, 10)
  line L6 (-99.6, 10) -> (-99.6, 20)
  line L7 (-99.6, 20) -> (-94.6, 20)
  line L8 (-94.6, 20) -> (-94.6, 17.3324)
  arc A1 (-81, 15) -> (-94.6, 17.3324) centre (-88, 15) ccw
  line L9 (-81, 15) -> (-81, 16)
  line L10 (-81, 16) -> (-37, 16)
  line L11 (-37, 16) -> (-37, 3)
  line L12 (-37, 3) -> (-81, 3)
  line L13 (-81, 3) -> (-81, 15)
  circle A2 centre (-72.5, 18.1) radius 1.625
  line L14 (-9.75, 10.558) -> (-33.75, 10.558)
  line L15 (-33.75, 10.558) -> (-33.75, 23.558)
  line L16 (-33.75, 23.558) -> (-9.75, 23.558)
  line L17 (-9.75, 23.558) -> (-9.75, 10.558)
  circle A3 centre (-33.5, 3.06) radius 1.5
  circle A4 centre (-33.5, 26.86) radius 1.5
  circle A5 centre (-10, 3.06) radius 1.5
  circle A6 centre (-10, 26.86) radius 1.5
  line L18 (-2, 20) -> (-2, 10)
  line L19 (-2, 10) -> (-7, 10)
  line L20 (-7, 10) -> (-7, 20)
  line L21 (-7, 20) -> (-2, 20)
  line L22 (1, 31) -> (-102.6, 31)
  line L23 (-102.6, 31) -> (-102.6, -1)
  line L24 (-102.6, -1) -> (1, -1)
  line L25 (1, -1) -> (1, 31)
  line L26 (-36.7, 29.3) -> (-36.7, 16.7)
  line L27 (-36.7, 16.7) -> (-58.3, 16.7)
  line L28 (-58.3, 16.7) -> (-58.3, 29.3)
  line L29 (-58.3, 29.3) -> (-36.7, 29.3)
  dimension "d398" = -0.8
extrude "Extrude54" add sketch "USB Holder" along normal blind 47 contours L26 L27 L28 L29 bodies 4
ref_plane "WorkPlane4" through (47.5, 57, 23) normal (0, 1, 0) x (0, 0, 1)
sketch "Knob1" plane through (47.5, 57, 23) normal (0, 1, 0) x (1, 0, 0)
  line L0 (10.8, -6.3) -> (10.8, 6.3)
  line L1 (-10.8, -6.3) -> (10.8, -6.3)
  line L2 (-10.8, 6.3) -> (-10.8, -6.3)
  line L3 (10.8, 6.3) -> (-10.8, 6.3)
  line L4 (-11.6, 7.1) -> (-11.6, -7.1)
  line L5 (-11.6, -7.1) -> (11.6, -7.1)
  line L6 (11.6, -7.1) -> (11.6, 7.1)
  line L7 (11.6, 7.1) -> (-11.6, 7.1)
  dimension "d402" = 0.8
extrude "Extrude55" add sketch "Knob1" along normal blind 5 separate body makes body 5
box "BoxPrimitive11" add length 14.2 width 23.2 height 0.8 placed x (0, 0, -1) y (-1, 0, 0) z (0, 1, 0) at (59.1, 62, 30.1) bodies 5
ref_plane "WorkPlane5" through (88, -6, 13.7919) normal (0, -1, 0) x (1, 0, 0)
sketch "Knob 2" plane through (88, -6, 13.7919) normal (0, -1, 0) x (1, 0, 0)
  line L0 (2.5981, 2.7081) -> (-2.5981, 2.7081)
  arc A0 (-2.5981, 2.7081) -> (2.5981, 2.7081) centre (0, 1.2081) ccw
  circle A1 centre (0, 1.2081) radius 11
  dimension "d411" = 22
  constraint concentric A0 A1
  measures "d411" diameter of A1
extrude "Extrude56" add sketch "Knob 2" along normal blind 5 separate body contours L0 A0 | A1 makes body 6
cylinder "CylinderPrimitive15" add diameter 12 height 6 placed x (1, 0, 0) y (0, 0, -1) z (0, 1, 0) at (88, -6, 15) bodies 6
sketch "knob 3" plane through (0, 0, 0) normal (0, 1, 0) x (-1, 0, 0)
  circle A0 centre (-88, 15) radius 6
  line L0 (-90.5981, 16.5) -> (-85.4019, 16.5)
  arc A1 (-90.5981, 16.5) -> (-85.4019, 16.5) centre (-88, 15) ccw
extrude "Extrude57" cut sketch "knob 3" against normal blind 5 contours L0 A1 bodies 6
sketch "LED Hole 2" plane through (0, -5, 0) normal (0, -1, 0) x (1, 0, 0)
  line L0 (0, 0) -> (101.6, 0)
  line L1 (101.6, 0) -> (101.6, 30)
  line L2 (101.6, 30) -> (0, 30)
  line L3 (0, 30) -> (0, 0)
  line L4 (37.5, 17.5) -> (37.5, 28.5)
  line L5 (37.5, 28.5) -> (57.5, 28.5)
  line L6 (57.5, 28.5) -> (57.5, 17.5)
  line L7 (57.5, 17.5) -> (37.5, 17.5)
  circle A0 centre (88, 15) radius 7
  circle A1 centre (72.5, 10.1) radius 3
  line L8 (36.25, 8.058) -> (7.25, 8.058)
  line L9 (7.25, 8.058) -> (7.25, 26.058)
  line L10 (7.25, 26.058) -> (36.25, 26.058)
  line L11 (36.25, 26.058) -> (36.25, 8.058)
  line L12 (40.25, 14.35) -> (54.75, 14.35)
  line L13 (54.75, 14.35) -> (54.75, 6.85)
  line L14 (54.75, 6.85) -> (40.25, 6.85)
  line L15 (40.25, 6.85) -> (40.25, 14.35)
  circle A2 centre (64.5, 10.1) radius 3
  circle A3 centre (72.5, 18.1) radius 2.625
  circle A4 centre (64.5, 18.1) radius 1.625
  dimension "d421" = 3.25
  measures "d421" diameter of A4
extrude "Extrude58" cut sketch "LED Hole 2" against normal blind 5 contours A4 bodies 4
chamfer "Chamfer12" distance 1 angle 45 1 edges at (62.985, -5, 18.6876) on bodies 4
chamfer "Chamfer13" distance 0.5 angle 45 4 edges at (40.25, -5, 10.6) (47.5, -5, 14.35) (54.75, -5, 10.6) (47.5, -5, 6.85) on bodies 4
chamfer "Chamfer14" distance 0.5 angle 45 4 edges at (57.5, -5, 23) (47.5, -5, 28.5) (37.5, -5, 23) (47.5, -5, 17.5) on bodies 4
sketch "Body Base" plane through (0, 0, 0) normal (0, 0, 1) x (1, 0, 0)
  line L0 (0, 0) -> (101.6, 0)
  line L1 (101.6, 0) -> (101.6, 110)
  line L2 (0, 110) -> (0, 0)
  line L3 (0, 110) -> (101.6, 110)
  circle A0 centre (3.8, 101) radius 1.5
  circle A1 centre (97.8, 99.0406) radius 1.5
  circle A2 centre (3.8, 31) radius 1.5
  circle A3 centre (97.8, 31) radius 1.5
  dimension "d427" = 101.6
  dimension "d432" = 3
  dimension "d433" = 3
  dimension "d434" = 3
  dimension "d435" = 3
  constraint horizontal L0
  constraint vertical L1
  constraint vertical L2
  constraint coincident L0.start L2.end
  constraint perpendicular L1 L3
  measures "d427" distance of L0.start L0.end
  measures "d432" diameter of A0
  measures "d433" diameter of A1
  measures "d434" diameter of A2
  measures "d435" diameter of A3
extrude "Extrude59" add sketch "Body Base" along normal blind 3 separate body makes body 7
box "BoxPrimitive12" add length 110 width 3 height 27 placed x (0, 1, 0) y (-1, 0, 0) z (0, 0, 1) at (101.6, 0, 3) bodies 7
box "BoxPrimitive13" add length 110 width 3 height 27 placed x (0, -1, 0) y (1, 0, 0) z (0, 0, 1) at (0, 110, 3) bodies 7
hole "Hole10" at (3.8, 31, 0) direction (0, 0, 1) diameter 3 depth 30 tip angle 180 bodies 7
hole "Hole11" at (97.8, 99.0406, 0) direction (0, 0, 1) diameter 3 depth 30 tip angle 180 bodies 7
hole "Hole12" at (97.8, 31, 0) direction (0, 0, 1) diameter 3 depth 30 tip angle 180 bodies 7
hole "Hole13" at (3.8, 101, 0) direction (0, 0, 1) diameter 3 depth 30 tip angle 180 bodies 7
move_face "OffsetFaces2" offset 10 1 faces at (66.7333, 110, 1) on bodies 7
move_face "OffsetFaces3" offset 20 1 faces at (66.7333, 120, 1) on bodies 7
sketch "Base Sides" plane through (101.6, 0, 0) normal (1, 0, 0) x (0, 1, 0)
  line L0 (0, 0) -> (140, 0)
  line L1 (140, 0) -> (140, 30)
  line L2 (140, 30) -> (0, 30)
  line L3 (0, 30) -> (0, 0)
  circle A0 centre (21, 5) radius 1.5
  circle A1 centre (111, 5) radius 1.5
  dimension "d464" = 90
  dimension "d465" = 3
  dimension "d466" = 3
  measures "d464" distance of A0.centre A1.centre
  measures "d465" diameter of A0
  measures "d466" diameter of A1
extrude "Extrude60" cut sketch "Base Sides" against normal blind 102 contours A0 | A1 bodies 7
move_face "OffsetFaces4" offset -19 1 faces at (66.7333, 140, 1) on bodies 7
sketch "Base Cutout" plane through (0, 0, 3) normal (0, 0, 1) x (-1, 0, 0)
  line L0 (-3, -99.7311) -> (-3, -32.2689)
  arc A0 (-3, -29.7311) -> (-3, -32.2689) centre (-3.8, -31) ccw
  line L1 (-3, -29.7311) -> (-3, 0)
  line L2 (-3, 0) -> (-98.6, 0)
  line L3 (-98.6, 0) -> (-98.6, -29.7311)
  arc A1 (-98.6, -32.2689) -> (-98.6, -29.7311) centre (-97.8, -31) ccw
  line L4 (-98.6, -32.2689) -> (-98.6, -97.7718)
  arc A2 (-98.6, -100.3095) -> (-98.6, -97.7718) centre (-97.8, -99.0406) ccw
  line L5 (-98.6, -100.3095) -> (-98.6, -121)
  line L6 (-98.6, -121) -> (-3, -121)
  line L7 (-3, -121) -> (-3, -102.2689)
  arc A3 (-3, -99.7311) -> (-3, -102.2689) centre (-3.8, -101) ccw
  line L8 (-14.9874, -121) -> (-14.9874, -105)
  line L9 (-79.9963, -121) -> (-79.9963, -105)
  line L10 (-79.9963, -105) -> (-14.9874, -105)
  constraint coincident L6 L8.start
  constraint perpendicular L6 L8
  constraint coincident L6 L9.start
  constraint perpendicular L6 L9
  constraint perpendicular L8 L10
extrude "Extrude61" cut sketch "Base Cutout" against normal blind 3 contours L6 L8 L9 L10 bodies 7
sketch "Base Mounts" plane through (0, 0, 3) normal (0, 0, 1) x (-1, 0, 0)
  line L0 (-79.9963, -121) -> (-79.9963, -105)
  line L1 (-79.9963, -105) -> (-14.9874, -105)
  line L2 (-14.9874, -105) -> (-14.9874, -121)
  line L3 (-14.9874, -121) -> (-3, -121)
  line L4 (-3, -121) -> (-3, -102.2689)
  arc A0 (-3, -99.7311) -> (-3, -102.2689) centre (-3.8, -101) ccw
  line L5 (-3, -99.7311) -> (-3, -32.2689)
  arc A1 (-3, -29.7311) -> (-3, -32.2689) centre (-3.8, -31) ccw
  line L6 (-3, -29.7311) -> (-3, 0)
  line L7 (-3, 0) -> (-98.6, 0)
  line L8 (-98.6, 0) -> (-98.6, -29.7311)
  arc A2 (-98.6, -32.2689) -> (-98.6, -29.7311) centre (-97.8, -31) ccw
  line L9 (-98.6, -32.2689) -> (-98.6, -97.7718)
  arc A3 (-98.6, -100.3095) -> (-98.6, -97.7718) centre (-97.8, -99.0406) ccw
  line L10 (-98.6, -100.3095) -> (-98.6, -121)
  line L11 (-98.6, -121) -> (-79.9963, -121)
  arc A4 (-3, -96.0644) -> (-3, -105.9356) centre (-3.8, -101) ccw
  arc A5 (-98.6, -103.9762) -> (-98.6, -94.1051) centre (-97.8, -99.0406) ccw
  arc A6 (-98.6, -35.9356) -> (-98.6, -26.0644) centre (-97.8, -31) ccw
  arc A7 (-3, -26.0644) -> (-3, -35.9356) centre (-3.8, -31) ccw
  dimension "d472" = 10
  dimension "d473" = 10
  dimension "d474" = 10
  dimension "d475" = 10
  constraint concentric A0 A4
  constraint coincident L4 A4.end
  constraint coincident L5 A4.start
  constraint concentric A3 A5
  constraint coincident L9 A5.end
  constraint coincident L10 A5.start
  constraint concentric A2 A6
  constraint coincident L8 A6.end
  constraint coincident L9 A6.start
  constraint concentric A1 A7
  constraint coincident L5 A7.end
  constraint coincident L6 A7.start
  measures "d472" diameter of A4
  measures "d473" diameter of A5
  measures "d474" diameter of A6
  measures "d475" diameter of A7
extrude "Extrude62" add sketch "Base Mounts" along normal blind 5 contours L9 A3 L10 A5 | L8 A2 L9 A6 | L4 A0 L5 A4 | L5 A1 L6 A7 bodies 7
sketch "Side Mounts L" plane through (3, 0, 0) normal (1, 0, 0) x (0, 1, 0)
  line L0 (96.0644, 8) -> (99.7311, 8)
  line L1 (99.7311, 8) -> (99.7311, 30)
  line L2 (99.7311, 30) -> (32.2689, 30)
  line L3 (32.2689, 30) -> (32.2689, 8)
  line L4 (32.2689, 8) -> (35.9356, 8)
  line L5 (35.9356, 8) -> (35.9356, 3)
  line L6 (35.9356, 3) -> (96.0644, 3)
  line L7 (96.0644, 3) -> (96.0644, 8)
  line L8 (35.9356, 3) -> (94.1051, 3)
  line L9 (103.9762, 3) -> (121, 3)
  line L10 (0, 3) -> (26.0644, 3)
  line L11 (25.5, 5) -> (25.5, 3)
  line L12 (16.5, 5) -> (16.5, 3)
  arc A0 (25.5, 5) -> (16.5, 5) centre (21, 5) ccw
  line L13 (16.5, 3) -> (25.5, 3)
  line L14 (106.5116, 5.3236) -> (106.5116, 3)
  line L15 (115.4914, 4.7212) -> (115.4914, 3)
  line L16 (106.5116, 3) -> (115.4914, 3)
  arc A1 (115.4914, 4.7212) -> (106.5116, 4.6764) centre (111, 5) ccw
  constraint tangent L11 A0
  constraint perpendicular L10 L11
  constraint coincident L10 L12.end
  constraint tangent L12 A0
  constraint perpendicular L10 L12
  constraint coincident L9 L14.end
  constraint perpendicular L9 L14
  constraint coincident L9 L15.end
  constraint perpendicular L9 L15
  constraint coincident L14 A1.end
extrude "Extrude63" add sketch "Side Mounts L" along normal blind 5 contours L9 L14 L15 L16 A1 | L10 L11 L12 A0 L13 bodies 7
hole "Hole14" at (0, 111, 5) direction (1, 0, 0) diameter 3 depth 13 tip angle 118 bodies 7
hole "Hole15" at (0, 21, 5) direction (1, 0, 0) diameter 3 depth 13 tip angle 118 bodies 7
sketch " Side Mounts R" plane through (98.6, 0, 0) normal (-1, 0, 0) x (0, -1, 0)
  line L0 (-97.7718, 8) -> (-94.1051, 8)
  line L1 (-94.1051, 8) -> (-94.1051, 3)
  line L2 (-94.1051, 3) -> (-35.9356, 3)
  line L3 (-35.9356, 3) -> (-35.9356, 8)
  line L4 (-35.9356, 8) -> (-32.2689, 8)
  line L5 (-32.2689, 8) -> (-32.2689, 30)
  line L6 (-32.2689, 30) -> (-97.7718, 30)
  line L7 (-97.7718, 30) -> (-97.7718, 8)
  circle A0 centre (-21, 5) radius 1.5
  arc A1 (-16.5, 5) -> (-25.5, 5) centre (-21, 5) ccw
  line L8 (-16.5, 5) -> (-16.5, 3)
  line L9 (-16.5, 3) -> (-25.5, 3)
  line L10 (-25.5, 3) -> (-25.5, 5)
  circle A2 centre (-111, 5) radius 1.5
  arc A3 (-106.5116, 5.3236) -> (-115.4914, 4.7212) centre (-111, 5) ccw
  line L11 (-106.5116, 5.3236) -> (-106.5116, 3)
  line L12 (-106.5116, 3) -> (-115.4914, 3)
  line L13 (-115.4914, 3) -> (-115.4914, 4.7212)
extrude "Extrude64" add sketch " Side Mounts R" along normal blind 4 contours A1 L8 L9 L10 | A3 L11 L12 L13 bodies 7
sketch "Encode Mount" plane through (0, 16, 0) normal (0, -1, 0) x (1, 0, 0)
  line L0 (87, 22) -> (82, 22)
  line L1 (82, 22) -> (82, 8)
  line L2 (82, 8) -> (94, 8)
  line L3 (94, 8) -> (94, 22)
  line L4 (94, 22) -> (89, 22)
  spline S0 degree 3 poles (89.5108, 18.0927) (89.7674, 17.9409) (90.0032, 17.7562) (90.4153, 17.334) (90.5912, 17.0994) (90.9393, 16.4773) (91.0724, 16.0738) (91.1723, 15.2519) (91.1433, 14.8421) (90.9311, 14.0707) (90.755, 13.7152) (90.2829, 13.1041) (89.9957, 12.8512) (89.6675, 12.6616) knots -0.655752 -0.655752 -0.655752 -0.655752 -0.566597 -0.566597 -0.479296 -0.479296 -0.35335 -0.35335 -0.231484 -0.231484 -0.1137 -0.1137 0 0 0 0
  arc A0 (86.3325, 12.6616) -> (89.6675, 12.6616) centre (88, 15) ccw
  spline S1 degree 3 poles (86.3325, 12.6616) (86.1126, 12.7886) (85.9106, 12.9444) (85.5475, 13.3084) (85.3891, 13.5162) (85.0611, 14.0869) (84.9333, 14.4679) (84.8267, 15.2711) (84.854, 15.6861) (85.0674, 16.4966) (85.2565, 16.8828) (85.7784, 17.5737) (86.1105, 17.8686) (86.4892, 18.0927) knots -0.658261 -0.658261 -0.658261 -0.658261 -0.581826 -0.581826 -0.503539 -0.503539 -0.383795 -0.383795 -0.259957 -0.259957 -0.132024 -0.132024 0 0 0 0
  line L5 (98.6, 30) -> (98.6, 3)
  line L6 (3, 3) -> (98.6, 3)
  line L7 (98.6, 3) -> (78.6, 3)
  line L8 (78.6, 3) -> (78.6, 26)
  line L9 (78.6, 26) -> (98.6, 26)
  line L10 (98.6, 26) -> (98.6, 3)
  line L11 (89, 21) -> (89, 22)
  line L12 (87, 22) -> (87, 21)
  circle A1 centre (88, 15) radius 3.5
  circle A2 centre (88, 21.5) radius 1.5
  dimension "d489" = 20
  dimension "d490" = 23
  dimension "d491" = 7
  dimension "d492" = 3
  constraint horizontal L7
  constraint vertical L8
  constraint horizontal L9
  constraint vertical L10
  constraint coincident L5.end L6.end
  measures "d489" distance of L5.end L7.end
  measures "d490" distance of L5.end L9.end
  measures "d491" diameter of A1
  measures "d492" diameter of A2
extrude "Extrude65" add sketch "Encode Mount" along normal blind 3 contours L0 L1 L2 L3 L4 A2 | L5 L6 L7 L8 L9 L10 bodies 7
sketch "Base 2" plane through (0, 0, 3) normal (0, 0, 1) x (-1, 0, 0)
  line L0 (-98.6, -13) -> (-78.6, -13)
  line L1 (-78.6, -13) -> (-78.6, -16)
  line L2 (-78.6, -16) -> (-98.6, -16)
  line L3 (-98.6, -16) -> (-98.6, -16.5)
  line L4 (-98.6, -16.5) -> (-94.6, -16.5)
  line L5 (-94.6, -16.5) -> (-94.6, -25.5)
  line L6 (-94.6, -25.5) -> (-98.6, -25.5)
  line L7 (-98.6, -25.5) -> (-98.6, -26.0644)
  arc A0 (-98.6, -35.9356) -> (-98.6, -26.0644) centre (-97.8, -31) ccw
  line L8 (-98.6, -35.9356) -> (-98.6, -94.1051)
  arc A1 (-98.6, -103.9762) -> (-98.6, -94.1051) centre (-97.8, -99.0406) ccw
  line L9 (-98.6, -103.9762) -> (-98.6, -106.5116)
  line L10 (-98.6, -106.5116) -> (-94.6, -106.5116)
  line L11 (-94.6, -106.5116) -> (-94.6, -115.4914)
  line L12 (-94.6, -115.4914) -> (-98.6, -115.4914)
  line L13 (-98.6, -115.4914) -> (-98.6, -121)
  line L14 (-98.6, -121) -> (-79.9963, -121)
  line L15 (-79.9963, -121) -> (-79.9963, -105)
  line L16 (-79.9963, -105) -> (-14.9874, -105)
  line L17 (-14.9874, -105) -> (-14.9874, -121)
  line L18 (-14.9874, -121) -> (-3, -121)
  line L19 (-3, -121) -> (-3, -115.4914)
  line L20 (-3, -115.4914) -> (-8, -115.4914)
  line L21 (-8, -115.4914) -> (-8, -106.5116)
  line L22 (-8, -106.5116) -> (-3, -106.5116)
  line L23 (-3, -106.5116) -> (-3, -105.9356)
  arc A2 (-3, -96.0644) -> (-3, -105.9356) centre (-3.8, -101) ccw
  line L24 (-3, -96.0644) -> (-3, -35.9356)
  arc A3 (-3, -26.0644) -> (-3, -35.9356) centre (-3.8, -31) ccw
  line L25 (-3, -26.0644) -> (-3, -25.5)
  line L26 (-3, -25.5) -> (-8, -25.5)
  line L27 (-8, -25.5) -> (-8, -16.5)
  line L28 (-8, -16.5) -> (-3, -16.5)
  line L29 (-3, -16.5) -> (-3, 0)
  line L30 (-3, 0) -> (-98.6, 0)
  line L31 (-98.6, 0) -> (-98.6, -13)
  circle A4 centre (-22.5, -84.5) radius 5
  circle A5 centre (-72.5, -84.5) radius 5
  circle A6 centre (-22.5, -63.5) radius 5
  circle A7 centre (-72.5, -63.5) radius 5
  circle A8 centre (-72.5, -13.5) radius 5
  dimension "d495" = 10
  dimension "d496" = 10
  dimension "d497" = 10
  dimension "d498" = 10
  dimension "d499" = 10
  measures "d495" diameter of A4
  measures "d496" diameter of A5
  measures "d497" diameter of A6
  measures "d498" diameter of A7
  measures "d499" diameter of A8
extrude "Extrude66" add sketch "Base 2" along normal blind 2 contours A4 | A5 | A6 | A7 | A8 bodies 7
hole "Hole16" at (22.5, 63.5, 5) direction (0, 0, -1) diameter 3 depth 13 tip angle 118 bodies 7
hole "Hole17" at (72.5, 63.5, 5) direction (0, 0, -1) diameter 3 depth 13 tip angle 118 bodies 7
hole "Hole18" at (72.5, 13.5, 5) direction (0, 0, -1) diameter 3 depth 13 tip angle 118 bodies 7
cylinder "CylinderPrimitive16" add diameter 2.75 height 3 placed x (1, 0, 0) y (0, 1, 0) z (0, 0, 1) at (22.5, 84.5, 5) bodies 7
cylinder "CylinderPrimitive17" add diameter 2.75 height 3 placed x (1, 0, 0) y (0, 1, 0) z (0, 0, 1) at (72.5, 84.5, 5) bodies 7
chamfer "Chamfer15" distance 1 angle 45 1 edges at (71.218, 84.0028, 8) on bodies 7
chamfer "Chamfer16" distance 1 angle 45 1 edges at (21.218, 84.0028, 8) on bodies 7
hole "Hole19" at (88, 13, 15) direction (0, 1, 0) diameter 8 depth 10 tip angle 118 bodies 7
box "BoxPrimitive14" cut length 10 width 11 height -7 placed x (0, 0, 1) y (0, -1, 0) z (1, 0, 0) at (99.6, 11, 10) bodies 4
box "BoxPrimitive15" cut length 11 width 11 height -8 placed x (0, 0, -1) y (0, -1, 0) z (-1, 0, 0) at (2, 11, 20) bodies 4